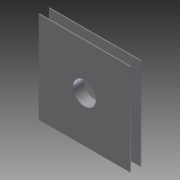
# Autodesk Inventor part: lazysusanbasic
Saved by Autodesk Inventor 2011 (Build 150239000, 239)
## iProperties
Created: 2011-07-30
Part Number: lazysusanbasic
Document SubType Name: Modeling
Designer: adowning
Density: 1 g/cm^3
Author: adowning
Autodesk Inventor part; units mm, degrees
ref_plane "YZ Plane" through (0, 0, 0) normal (1, 0, 0) x (0, 1, 0)
ref_plane "XZ Plane" through (0, 0, 0) normal (0, 1, 0) x (-1, 0, 0)
ref_plane "XY Plane" through (0, 0, 0) normal (0, 0, 1) x (1, 0, 0)
sketch "Sketch1" plane through (0, 0, 0) normal (0, 0, 1) x (1, 0, 0)
  line L0 (-24.746, 21.5893) -> (76.854, 21.5893)
  line L1 (76.854, 21.5893) -> (76.854, -80.0107)
  line L2 (76.854, -80.0107) -> (-24.746, -80.0107)
  line L3 (-24.746, -80.0107) -> (-24.746, 21.5893)
  line L4 (-24.746, 21.5893) -> (76.854, -80.0107)
  line L5 (76.854, 21.5893) -> (-24.746, -80.0107)
  circle A0 centre (26.054, -29.2107) radius 12.7
  point P0 (0, 0)
  dimension "d0" = 101.6
  dimension "d1" = 101.6
  dimension "d2" = 25.4
  constraints: 12 end point, 2 parallel, 1 centre point, 1 horizontal, 1 midpoint, 1 perpendicular
  measures "d0" distance of L1.end L2.end
  measures "d1" distance of L0.end L1.end
  measures "d2" diameter of A0
extrude "Extrusion1" add sketch "Sketch1" along normal blind 8.128 and the other way blind 3.937
sketch "Sketch2" plane through (0, 0, 8.128) normal (0, 0, 1) x (1, 0, 0)
  line L0 (-24.746, 21.5893) -> (76.854, -80.0107)
  line L1 (76.854, 21.5893) -> (-24.746, -80.0107)
  circle A0 centre (26.054, -29.2107) radius 12.7
  point P0 (0, 0)
  dimension "d7" = 25.4
  constraints: 4 end point, 2 midpoint, 1 centre point, 1 perpendicular
  measures "d7" diameter of A0
extrude "Extrusion2" cut sketch "Sketch2" against normal blind 8.128
sketch "Sketch3" plane through (-24.746, 21.5893, 8.128) normal (0, 1, 0) x (1, 0, 0)
  line L0 (101.6, 12.065) -> (101.6, 0) projected
  line L1 (101.6, 12.065) -> (0, 12.065) projected
  line L2 (0, 0) -> (0, 12.065) projected
  line L3 (0, 12.065) -> (101.6, 12.065)
  line L4 (101.6, 12.065) -> (101.6, 11.303)
  line L5 (101.6, 11.303) -> (0, 11.303)
  line L6 (0, 11.303) -> (0, 12.065)
  line L7 (101.6, 0) -> (0, 0)
  line L8 (0, 0) -> (0, 0.762)
  line L9 (0, 0.762) -> (101.6, 0.762)
  line L10 (101.6, 0.762) -> (101.6, 0)
  line L11 (0, 0.762) -> (0, 11.303)
  line L12 (101.6, 12.065) -> (101.6, 0.762)
  point P0 (24.746, 8.128)
  dimension "d10" = 0.762
  dimension "d11" = 0.762
  constraints: 20 end point, 4 parallel, 3 perpendicular, 2 horizontal, 2 point on line, 1 collinear
  measures "d10" distance of L3.end L4.end
  measures "d11" distance of L7.end L8.end
extrude "Extrusion3" cut sketch "Sketch3" against normal blind 101.6 contours L0 L9 L2 L5
sketch "Sketch4" plane through (0, 0, 8.128) normal (0, 0, 1) x (1, 0, 0)
  circle A0 centre (26.054, -29.2107) radius 12.7 projected
  circle A1 centre (26.054, -29.2107) radius 19.05
  point P0 (0, 0)
  dimension "d14" = 38.1
  constraints: 1 centre point, 1 coincident
  measures "d14" diameter of A1
extrude "Extrusion4" add sketch "Sketch4" against normal blind 8.128
sketch "Sketch5" plane through (0, 0, 8.128) normal (0, 0, 1) x (1, 0, 0)
  circle A0 centre (26.054, -29.2107) radius 12.7 projected
  point P0 (0, 0)
extrude "Extrusion5" cut sketch "Sketch5" against normal blind 25.4
sketch "Sketch6" plane through (26.054, -29.2107, 0) normal (0, 0, -1) x (-1, 0, 0)
  circle A0 centre (0, 0) radius 12.7 projected
  circle A1 centre (0, 0) radius 19.05 projected
  point P0 (26.054, 29.2107)
extrude "Extrusion6" add sketch "Sketch6" along normal blind 3.556
body "Solid1"
